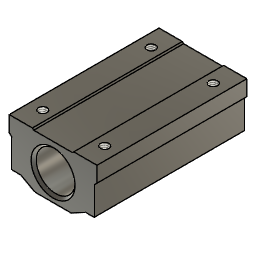
Slider block D15 v1 (Autodesk Fusion 360 design; units mm, degrees)
Autodesk Fusion 360 part; units mm, degrees
sketch "Sketch1" plane through (0, 0, 0) normal (0, 1, 0) x (1, 0, 0)
  circle A0 centre (0, 0) radius 7.5
  line L0 (-17, -11) -> (17, -11)
  line L1 (17, -11) -> (17, -5)
  line L2 (17, -5) -> (16, -4)
  line L3 (16, -4) -> (16, 7)
  line L4 (16, 7) -> (12.5, 7)
  line L5 (12.5, 7) -> (7, 10)
  line L6 (-17, -11) -> (-17, -5)
  line L7 (-17, -5) -> (-16, -4)
  line L8 (-16, -4) -> (-16, 7)
  line L9 (-16, 7) -> (-12.5, 7)
  line L10 (-12.5, 7) -> (-7, 10)
  line L11 (-7, 10) -> (7, 10)
  dimension "d1" = 15
  dimension "d2" = 34
  dimension "d3" = 14
  dimension "d4" = 21
  constraint coincident A0.centre origin
  constraint perpendicular L0 L1
  constraint perpendicular L3 L4
  constraint perpendicular L0 L6
  constraint perpendicular L8 L9
  constraint horizontal L11
  constraint equal L1 L6
  constraint equal L3 L8
  constraint equal L4 L9
  constraint equal L5 L10
  constraint equal L2 L7
  measures "d1" diameter of A0
  measures "d2" distance of L0.start L0.end
  measures "d3" distance of L5.end L10.end
  measures "d4" distance of L0 L11
extrude "Extrude1" add sketch "Sketch1" along normal mid plane 58
sketch "Sketch2" plane through (0, 0, 11) normal (0, 0, 1) x (-1, 0, 0)
  line L0 (-17, 29) -> (-17, -29)
  line L1 (-17, -29) -> (17, -29)
  line L2 (17, -29) -> (17, 29)
  line L3 (17, 29) -> (-17, 29)
  line L4 (0, -21) -> (0, 21) construction
  line L5 (17, 0) -> (-17, 0) construction
  line L6 (-12, -21) -> (12, -21) construction
  line L7 (12, 21) -> (-12, 21) construction
  circle A0 centre (-12, -21) radius 2
  circle A1 centre (-12, 21) radius 2
  circle A2 centre (12, 21) radius 2
  circle A3 centre (12, -21) radius 2
  line L8 (8, -29) -> (8, 29)
  line L9 (-10, -21) -> (-8, -21)
  line L10 (-8, -29) -> (-8, 29)
  dimension "d7" = 42
  dimension "d8" = 24
  dimension "d13" = 16
  constraint vertical L4
  constraint midpoint L2 L5.start
  constraint midpoint L0 L5.end
  constraint midpoint L4 L5
  constraint perpendicular L4 L6
  constraint perpendicular L4 L7
  constraint coincident L6.start A0.centre
  constraint coincident L7.end A1.centre
  constraint coincident L7.start A2.centre
  constraint coincident L6.end A3.centre
  constraint coincident L1 L8.start
  constraint coincident L3 L8.end
  constraint perpendicular L3 L8
  constraint coincident A0 L9.start
  constraint coincident L6 L9.start
  constraint coincident L6 L9.end
  constraint perpendicular L8 L9
  constraint coincident L1 L10.start
  constraint coincident L3 L10.end
  constraint perpendicular L3 L10
  measures "d7" distance of L4.start L4.end
  measures "d8" distance of L6.start L6.end
  measures "d13" distance of L8 L10
hole "Hole1" at (12, 21, 11) at (-12, 21, 11) at (-12, -21, 11) at (12, -21, 11) direction (0, 0, -1) diameter 3.332 depth 8 tip angle 118
thread "Thread1" "ISO Metric profile 4.0 M4x0.7 6H"
chamfer "Chamfer1" distance 1 angle 45 2 edges at (-6.9925, -29, 2.7121) (-6.9925, 29, -2.7121)
extrude "Extrude2" cut sketch "Sketch2" against normal blind 0.5 contours L1 L3 L8 L10
chamfer "Chamfer2" distance 0.5 angle 45 2 edges at (-8, 0, 10.5) (8, 0, 10.5)
fillet "Fillet1" radius 0.1 2 edges at (16, 0, -7) (-16, 0, -7)
